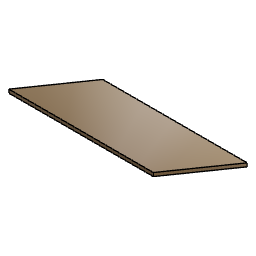
top_panel (Autodesk Fusion 360 design; units mm, degrees)
Autodesk Fusion 360 part; units mm, degrees
sketch "Top Panel" plane through (0, 0, 0) normal (1, 0, 0) x (0, 1, 0)
  line L0 (-0.0158, 146.1836) -> (175.2958, 74.2831)
  line L1 (175.2958, 80.7681) -> (-0.0158, 152.6686)
  line L2 (-0.0158, 152.6686) -> (-0.0158, 146.1836)
  line L3 (175.2958, 80.7681) -> (175.2958, 74.2831)
  dimension "d12" = 189.483
  dimension "d13" = 189.483
  dimension "d14" = 6
  dimension "d18" = 67.7
  constraint vertical L2
  constraint parallel L2 L3
  measures "d12" distance of L1.start L1.end
  measures "d13" distance of L0.start L0.end
  measures "d14" distance of L0 L1
  measures "d18" angle of L0 L3
extrude "Extrude2" add sketch "Top Panel" along normal blind 270
equation "MDFThickness = 6 mm" comment "Thickness of the MDF board"
equation "topPlateWidth = 210 mm" comment "Width of the top plate"
equation "baseBreadth = 250 mm" comment "Breadth of the base plate"
equation "filletRadius = 8 mm" comment "Radius of the side plate fillets"
named bodies: "Top Panel"
